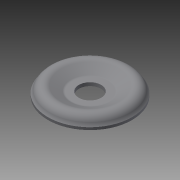
# Autodesk Inventor part: 2SS-UR
Saved by Autodesk Inventor 2014 SP2 (Build 180246200, 246)
## iProperties
Created: 2018-12-09
Part Number: 2SS-UR
Material: Generic
Catalog Web Link: www.cadenas.de
Description: 2 Series Stainless Steel Upper Race-Capacitiy up to 325 lbs Each
Vendor: COLSONGROUP
Document SubType Name: Modeling
Designer: psadmin
Manufacturer: COLSONGROUP
Mass: 10.5163 g
Surface Area: 82.373 cm^2
Volume: 10.5163 cm^3
Density: 1 g/cm^3
Appearance: PSOLRGB-175-175-175
Category: PARTsolutions
Company: COLSONGROUP
Title: 2SS-UR
Author: Cadenas PARTsolutions
Comments: Capacitiy up to 325 lbs Each
PSOL_IDENT_0: {$CADENAS_DATA\23d-libs\colsongroup\colson\casters\2_series_stainless_steel\2_series_stainless_steel
PSOL_IDENT_1: _upper_race.prj},181 {VTYP=3D},{NB=2SS-UR},{LINA=2SS-UR},{NN=2 Series Stainless Steel Upper Race},{D
PSOL_IDENT_2: ATE=13.07.2017 07:15:59},{GEOMDATE=03.02.2017 08:30:00},{VERSION=},{LINEID=40},{WBVAR=},{WBNUMERIC=}
PSOL_IDENT_3: {NB=2SS-UR},{LINA=2SS-UR},{KT=DUMMY},{PN=2SS-UR}
NN: 2 Series Stainless Steel Upper Race
NT: Capacitiy up to 325 lbs Each
NB: 2SS-UR
NBSYN: $PN.
LINA: 2SS-UR
PN: 2SS-UR
SUPPLIER: COLSONGROUP
ARTICLENO: 2SS-UR
BOMINFO: 2SS-UR
CREATOR: CADENAS GmbH
Autodesk Inventor part; units mm, degrees
sketch "Sketch_1" plane through (0, 0, 0) normal (0, 0, 1) x (1, 0, 0)
  line L0 (0, -6.731) -> (0, 0)
  line L1 (7.874, -6.731) -> (13.1064, -6.731)
  arc A0 (13.1064, -6.731) -> (15.3507, -6.2225) centre (13.1064, -1.524) ccw
  line L2 (15.3507, -6.2225) -> (22.0933, -3.0019)
  arc A1 (26.4708, -4.2657) -> (22.0933, -3.0019) centre (23.5712, -6.096) ccw
  arc A2 (26.4708, -4.2657) -> (28.3656, -7.2644) centre (36.703, 0.1016) ccw
  line L3 (28.3656, -7.2644) -> (30.3784, -7.2644)
  line L4 (30.3784, -7.2644) -> (30.3784, -5.4762)
  arc A3 (28.9785, -3.2814) -> (30.3784, -5.4762) centre (36.703, 0.1016) ccw
  arc A4 (28.9785, -3.2814) -> (20.7706, -0.6814) centre (23.5712, -6.096) ccw
  line L5 (20.7706, -0.6814) -> (13.9939, -4.1865)
  arc A5 (12.827, -4.4704) -> (13.9939, -4.1865) centre (12.827, -1.9304) ccw
  line L6 (12.827, -4.4704) -> (8.0718, -4.4704)
  line L7 (8.0718, -4.4704) -> (7.874, -6.731)
  constraints: 16 end point, 12 point on circle, 6 centre point
revolve "Revolution1" add sketch "Sketch_1" angle 360 about axis through (0, -6.731, 0) along (0, -1, 0)
sketch "Sketch_2" plane through (0, 0, 0) normal (0, 0, 1) x (1, 0, 0)
  line L0 (0, -12.7) -> (0, 12.7)
  circle A0 centre (23.368, -4.826) radius 2.286
  constraints: 2 end point, 1 centre point
revolve "Revolution2" add sketch "Sketch_2" angle 360 about axis through (0, -12.7, 0) along (0, -1, 0)
ref_plane "to_top_plate_XY" through (0, 0, 0) normal (0, -1, 0) x (1, 0, 0)
ref_plane "to_top_plate_YZ" through (0, 0, 0) normal (1, 0, 0) x (0, 0, 1)
ref_plane "to_top_plate_ZX" through (0, 0, 0) normal (0, 0, 1) x (0, -1, 0)
ref_plane "upper_race_XY" through (0, -6.731, 0) normal (0, 1, 0) x (1, 0, 0)
ref_plane "upper_race_YZ" through (0, -6.731, 0) normal (1, 0, 0) x (0, 0, -1)
ref_plane "upper_race_ZX" through (0, -6.731, 0) normal (0, 0, -1) x (0, 1, 0)
body "Solid1"
